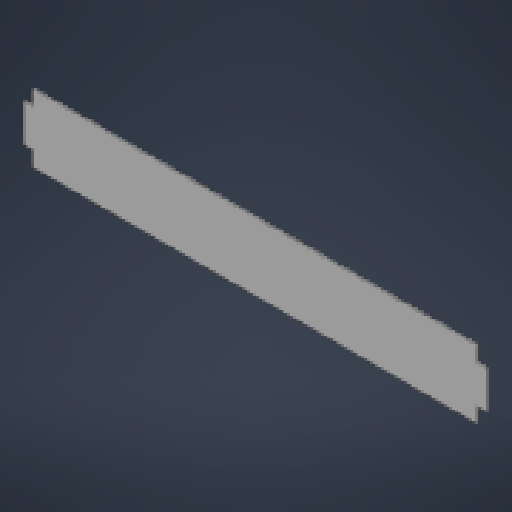
# Autodesk Inventor part: 内板
Saved by Autodesk Inventor 2025 (Build 290162000, 162)
## iProperties
Created: 2025-06-18
Part Number: 内板
Material: 常规
Document SubType Name: Modeling
Designer: XH
Density: 1 g/cm^3
Appearance: 默认
Author: XH
Autodesk Inventor part; units mm, degrees
ref_plane "YZ Plane" through (0, 0, 0) normal (1, 0, 0) x (0, 1, 0)
ref_plane "XZ Plane" through (0, 0, 0) normal (0, 1, 0) x (-1, 0, 0)
ref_plane "XY Plane" through (0, 0, 0) normal (0, 0, 1) x (1, 0, 0)
sketch "草图1" plane through (0, 0, 0) normal (0, 0, 1) x (1, 0, 0)
  line L0 (477.5, -70) -> (-477.5, -70)
  line L1 (-477.5, -70) -> (-477.5, 70)
  line L2 (-477.5, 70) -> (477.5, 70)
  line L3 (477.5, 70) -> (477.5, -70)
  line L4 (477.5, -70) -> (-477.5, 70) construction
  line L5 (-477.5, -70) -> (477.5, 70) construction
  line L6 (477.5, -40) -> (-477.5, -40) projected
  line L7 (477.5, 40) -> (-477.5, 40) projected
  line L8 (-457.5, 40) -> (-457.5, -40)
  line L9 (457.5, 40) -> (457.5, -40) projected
  line L10 (-455.5, -70) -> (-455.5, 70)
  line L11 (-475.5, 69.7068) -> (-475.5, -70)
  line L12 (475.5, 70) -> (475.5, -70)
  line L13 (455.5, 70) -> (455.5, -70)
  line L14 (475.5, -45) -> (-475.5, -45)
  line L15 (-475.5, -45) -> (-475.5, 45)
  line L16 (-475.5, 45) -> (475.5, 45)
  line L17 (475.5, 45) -> (475.5, -45)
  line L18 (475.5, -45) -> (-475.5, 45) construction
  line L19 (-475.5, -45) -> (475.5, 45) construction
  point P0 (0, 0)
  point P1 (457.5, -70)
  point P2 (457.5, 70)
  point P3 (-455.5, 40)
  point P4 (-455.5, -40)
  point P5 (475.5, -64)
  point P6 (475.5, 64)
  point P7 (-475.5, 40)
  point P8 (-475.5, -40)
  point P9 (455.5, -40)
  point P10 (475.5, -40)
  point P11 (475.5, 40)
  point P12 (455.5, 40)
  dimension "d0" = 140
  dimension "d1" = 955
  dimension "d6" = 2
  dimension "d7" = 2
  dimension "d8" = 2
  dimension "d9" = 2
  dimension "d12" = 90
  constraints: 34 end point, 14 point on line, 6 perpendicular, 4 midpoint, 4 parallel, 2 horizontal
  measures "d0" distance of L0.end L1.end
  measures "d1" distance of L1.end L2.end
  measures "d6" distance between parallel lines of L1 L11
  measures "d7" distance between parallel lines of L12 L3
  measures "d8" distance between parallel lines of L8 L10
  measures "d9" distance between parallel lines of L13 L9
  measures "d12" distance between parallel lines of L14 L16
extrude "拉伸1" add sketch "草图1" along normal blind 3 contours L0 L10 L14 L13 | L6 L9 L7 L12 | L14 L10 L6 L13 | L6 L13 L7 L9 | L6 L10 L7 L13 | L6 L8 L7 L10 | L7 L10 L16 L13 | L13 L16 L10 L2 | L11 L7 L8 L6
